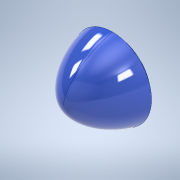
# Autodesk Inventor part: nose
Saved by Autodesk Inventor 2020 (Build 240168000, 168)
## iProperties
Created: 2021-01-23
Part Number: nose
Material: ABS Plastic
Document SubType Name: Modeling
Designer: 0x6f736f646f
Density: 1.06 g/cm^3
Appearance: Smooth - White
Author: 0x6f736f646f
Autodesk Inventor part; units mm, degrees
ref_plane "YZ Plane" through (0, 0, 0) normal (1, 0, 0) x (0, 1, 0)
ref_plane "XZ Plane" through (0, 0, 0) normal (0, 1, 0) x (-1, 0, 0)
ref_plane "XY Plane" through (0, 0, 0) normal (0, 0, 1) x (1, 0, 0)
sketch "Sketch1" plane through (0, 0, 0) normal (1, 0, 0) x (0, 1, 0)
  line L0 (0, 50) -> (13.2351, 50) construction
  line L1 (13.2351, 50) -> (33.2639, 29.3144) construction
  line L2 (33.2639, 29.3144) -> (40, 0) construction
  spline S0 degree 3 poles (0, 50) (13.2351, 50) (33.2639, 29.3144) (40, 0) knots 1 1 1 1 2 2 2 2
  line L3 (40, 0) -> (35, 0)
  line L4 (35, 0) -> (35, -4)
  line L5 (35, -4) -> (30, -4)
  line L6 (30, -4) -> (30, 0)
  line L7 (30, 0) -> (29.7058, 0)
  line L8 (0, 40) -> (0, 50)
  line L9 (0, -16.1106) -> (0, 68.6634) projected
  spline S1 degree 5 poles (0, 40) (0.4135, 39.9988) (0.8249, 39.9282) (1.2279, 39.838) (2.3939, 39.4976) (3.5072, 39.0068) (4.221, 38.6438) (5.8893, 37.6934) (7.4605, 36.5875) (8.3476, 35.9041) (10.2633, 34.3092) (12.0546, 32.575) (13.0069, 31.5853) (14.981, 29.3968) (16.811, 27.086) (17.7494, 25.8217) (19.6416, 23.1088) (21.3701, 20.2884) (22.2321, 18.7841) (23.9288, 15.6164) (25.4392, 12.3555) (26.1713, 10.6453) (27.4042, 7.5179) (28.4728, 4.3311) (28.9171, 2.8968) (29.3282, 1.4528) (29.7058, 0) knots 0 0 0 0 0 0 0.039846 0.039846 0.039846 0.11695 0.11695 0.11695 0.224832 0.224832 0.224832 0.357168 0.357168 0.357168 0.508897 0.508897 0.508897 0.675984 0.675984 0.675984 0.855263 0.855263 0.855263 1 1 1 1 1 1
  dimension "d51" = 10
  dimension "d45" = 5
  dimension "d46" = 4
  dimension "d47" = 5
  dimension "d49" = 30
  dimension "d50" = 40
  constraints: 12 end point, 3 perpendicular, 2 point on line, 1 horizontal, 1 vertical, 7 other
  measures "d45" distance of L2.end L3.end
  measures "d46" distance of L3.end L4.end
  measures "d47" distance of L4.end L5.end
  measures "d49" distance between parallel lines of L9 L6
  measures "d50" vertical distance of L7.end point (0, 40)
revolve "Revolution3" add sketch "Sketch1" angle 360 about axis through (0, 0, -10) along (0, 0, 1)
body "Solid2"
